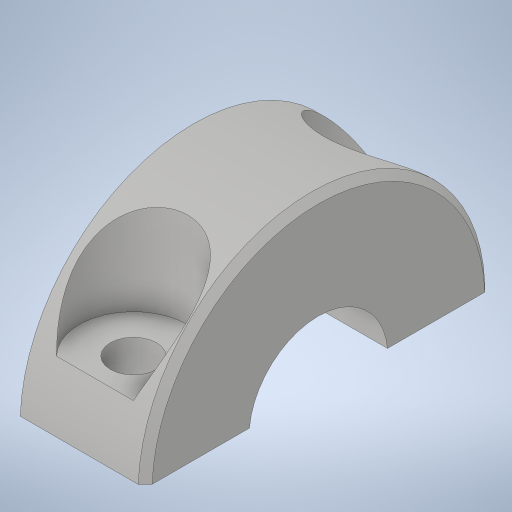
# Autodesk Inventor part: MBRDAC45-2-10_p2
Saved by Autodesk Inventor 2024 (Build 280153000, 153)
## iProperties
Created: 2024-03-05
Part Number: MBRDAC45-2-10_p2
Material: Generic
Catalog Web Link: www.cadenas.de
Description: MBRDC, MBRDAC_part2-Pulleys for Round Belts - Clamping Type - Trapezoid Groove
Vendor: MISUMI
Document SubType Name: Modeling
Designer: psAdmin
Manufacturer: MISUMI
Mass: 1.27874 g
Surface Area: 11.8178 cm^2
Volume: 1.27874 cm^3
Density: 1 g/cm^3
Appearance: PSOLRGB-175-175-175
Category: PARTsolutions
Company: MISUMI
PSOL_IDENT_0: {$CADENAS_DATA/23d-libs/misumi/metric/52_belts_pulleys/mbrdc/mbrdc_part2.prj},198 {VTYP=3D},{NB=MBRD
PSOL_IDENT_1: AC45-2-10_p2},{LINA=MBRDAC45-2-10},{NN=MBRDC, MBRDAC_part2},{DATE=06.06.2021 23:11:25},{GEOMDATE=10.
PSOL_IDENT_2: 06.2016 05:41:00},{VERSION=},{LINEID=30},{WBVAR=MAT,PD,DDS},{WBNUMERIC=PD,DDS}  {NB=MBRDAC45-2-10_p2
PSOL_IDENT_3: },{LINA=MBRDAC45-2-10},{KT=DUMMY},{PN=MBRDAC45-2-10},{TYPE=MBRDAC},{MAT=2},{ST=Clear Anodizing},{AC=
PSOL_IDENT_4: Hexagon Socket Head Cap Screw (x2) Stainless Steel},{PD=45},{PD0=23,28,30,40,45,48,60,80},{U=2.0},{D
PSOL_IDENT_5: DS=10.00},{DS0=5,6,6.35,8,10,11,12},{D=25},{D1=47},{D2=41},{HH=2.0},{W=4.4},{L=20},{T=10},{LL=4.5},{
PSOL_IDENT_6: X=9.0},{Y=4.5},{M=M4},{CBD=4},{MM=4.000},{MMMIN=3.242},{DD1=8.0},{DD2=4.5}
NB: MBRDAC45-2-10_p2
NN: MBRDC, MBRDAC_part2
NT: Pulleys for Round Belts - Clamping Type - Trapezoid Groove
NBSYN: $PN._p2
LINA: MBRDAC45-2-10
CATALOG: Misumi
PN: MBRDAC45-2-10
MAT: 5052 Aluminum Alloy
ST: Clear Anodizing
AC: Hexagon Socket Head Cap Screw (x2) Stainless Steel
PD: 45
U: 2
DDS: 10
D: 25
D1: 47
D2: 41
HH: 2
W: 4.4
L: 20
T: 10
LL: 4.5
X: 9
Y: 4.5
M: M4
CBD: 4
SUPPLIER: MISUMI
ARTICLENO: MBRDAC45-2-10_p2
BOMINFO: MBRDAC45-2-10
CREATOR: CADENAS GmbH
Title: MBRDAC45-2-10
Author: Cadenas PARTsolutions
Comments: Pulleys for Round Belts - Clamping Type - Trapezoid Groove
Autodesk Inventor part; units mm, degrees
sketch "Sketch_1" plane through (0, 0, 0) normal (0, 0, 1) x (1, 0, 0)
  line L0 (10.2, 0) -> (0, 0)
  line L1 (1.02, 5.1) -> (10.2, 5.1)
  line L2 (10.2, 5.1) -> (10.2, 12.24)
  line L3 (10.2, 12.24) -> (9.69, 12.75)
  line L4 (9.69, 12.75) -> (1.02, 12.75)
  line L5 (1.02, 12.75) -> (1.02, 5.1)
  dimension "d15" = 5.1
  constraints: 12 end point
  measures "d15" distance between parallel lines of L0 L1
revolve "Revolution1" add sketch "Sketch_1" angle 180 mid plane about axis through (10.2, 0, 0) along (-1, 0, 0)
sketch "Sketch_2" plane through (0, 0, 0) normal (0, 0, 1) x (1, 0, 0)
  line L0 (0, 0.5) -> (0, 0)
  line L1 (0, 0) -> (20, 0)
  line L2 (20, 0) -> (20, 0.5)
  line L3 (20, 0.5) -> (0, 0.5)
  constraints: 8 end point
extrude "Extrusion1" cut sketch "Sketch_2" along normal mid plane 50
ref_plane "part2_to_part1_XY" through (0, 0, 0) normal (1, 0, 0) x (0, 0, -1)
ref_plane "part2_to_part1_YZ" through (0, 0, 0) normal (0, 0, -1) x (0, 1, 0)
ref_plane "part2_to_part1_ZX" through (0, 0, 0) normal (0, 1, 0) x (1, 0, 0)
ref_plane "part2_to_screw1_XY" through (5.5, 4.5, 9) normal (0, 1, 0) x (1, 0, 0)
ref_plane "part2_to_screw1_YZ" through (5.5, 4.5, 9) normal (1, 0, 0) x (0, 0, -1)
ref_plane "part2_to_screw1_ZX" through (5.5, 4.5, 9) normal (0, 0, -1) x (0, 1, 0)
ref_plane "part2_to_screw2_XY" through (5.5, 4.5, -9) normal (0, 1, 0) x (1, 0, 0)
ref_plane "part2_to_screw2_YZ" through (5.5, 4.5, -9) normal (1, 0, 0) x (0, 0, -1)
ref_plane "part2_to_screw2_ZX" through (5.5, 4.5, -9) normal (0, 0, -1) x (0, 1, 0)
ref_plane "作業平面10" through (5.355, 12.75, 0) normal (0, 1, 0) x (-1, 0, 0)
sketch "スケッチ6" plane through (5.355, 12.75, 0) normal (0, 1, 0) x (-1, 0, 0)
  circle A0 centre (-0.25, -9) radius 2.25 projected
  circle A1 centre (-0.25, -9) radius 4
  circle A2 centre (-0.25, -9) radius 1.7
  circle A3 centre (-0.25, 9) radius 2.25 projected
  circle A4 centre (-0.25, 9) radius 4
  circle A5 centre (-0.25, 9) radius 1.7
  point P0 (5.355, 0)
  dimension "d7" = 8
  dimension "d8" = 3.4
  dimension "d9" = 8
  dimension "d10" = 3.4
  constraints: 4 centre point, 4 coincident
  measures "d7" diameter of A1
  measures "d8" diameter of A2
  measures "d9" diameter of A4
  measures "d10" diameter of A5
extrude "押し出し2" cut sketch "スケッチ6" against normal through all contours A2 | A5
extrude "押し出し3" cut sketch "スケッチ6" against normal blind 8 contours A0 | A1 | A2 | A3 | A4 | A5
body "Solid1"
